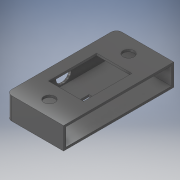
# Autodesk Inventor part: prototype1_third_eye_not_blind
Saved by Autodesk Inventor 2019 (Build 230136000, 136)
## iProperties
Created: 2019-02-05
Part Number: prototype1_third_eye_not_blind
Material: Generic
Document SubType Name: Modeling
Designer: ybharatu
Density: 1 g/cm^3
Appearance: Silicon Nitride - Polished
Author: ybharatu
Autodesk Inventor part; units mm, degrees
ref_plane "YZ Plane" through (0, 0, 0) normal (1, 0, 0) x (0, 1, 0)
ref_plane "XZ Plane" through (0, 0, 0) normal (0, 1, 0) x (-1, 0, 0)
ref_plane "XY Plane" through (0, 0, 0) normal (0, 0, 1) x (1, 0, 0)
sketch "Sketch1" plane through (0, 0, 0) normal (0, 1, 0) x (-1, 0, 0)
  line L0 (122.8458, -138.2757) -> (56.882, -138.2757)
  line L1 (56.882, -138.2757) -> (56.882, -265.2757)
  line L2 (56.882, -265.2757) -> (122.8458, -265.2757)
  line L3 (122.8458, -265.2757) -> (122.8458, -138.2757)
  line L4 (110.1458, -173.9373) -> (69.582, -173.9373)
  line L5 (69.582, -173.9373) -> (69.582, -229.6141)
  line L6 (69.582, -229.6141) -> (110.1458, -229.6141)
  line L7 (110.1458, -229.6141) -> (110.1458, -173.9373)
  point P0 (0, 0)
  dimension "d1" = 127
  dimension "d4" = 55.6768
  dimension "d5" = 40.5638
  dimension "d6" = 12.7
  dimension "d7" = 35.6616
  dimension "d8" = 12.7
  constraints: 16 end point, 4 parallel, 2 horizontal, 2 perpendicular
  measures "d1" distance of L2.end L0.start
  measures "d4" distance of L6.end L4.start
  measures "d5" distance of L5.end L6.end
  measures "d6" distance between parallel lines of L3 L7
  measures "d7" distance between parallel lines of L0 L4
  measures "d8" distance between parallel lines of L5 L1
extrude "Extrusion1" add sketch "Sketch1" along normal blind 25.4 contours L3 L2 L1 L0 | L7 L6 L5 L4
shell "Shell1" thickness 2.54 removed faces 1 at (-56.882, 8.4667, -180.609)
sketch "Sketch3" plane through (0, 25.4, 0) normal (0, 1, 0) x (1, 0, 0)
  line L0 (-110.1458, 174.0389) -> (-69.582, 174.0389)
  line L1 (-69.582, 174.0389) -> (-69.582, 229.7157)
  line L2 (-69.582, 229.7157) -> (-110.1458, 229.7157)
  line L3 (-110.1458, 229.7157) -> (-110.1458, 174.0389)
  line L4 (-122.8458, 265.2757) -> (-122.8458, 138.2757) projected
  line L5 (-56.882, 265.2757) -> (-122.8458, 265.2757) projected
  point P0 (0, 0)
  dimension "d14" = 55.6768
  dimension "d15" = 40.5638
  dimension "d16" = 12.7
  dimension "d17" = 35.56
  constraints: 8 end point, 2 parallel, 1 horizontal, 1 perpendicular
  measures "d14" distance of L2.end L0.start
  measures "d15" distance of L0.start L0.end
  measures "d16" distance between parallel lines of L4 L3
  measures "d17" distance between parallel lines of L5 L2
extrude "Extrusion2" cut sketch "Sketch3" against normal blind 12.7
sketch "Sketch4" plane through (0, 25.4, 0) normal (0, 1, 0) x (1, 0, 0)
  circle A0 centre (-91.0958, 156.2589) radius 6.35
  line L0 (-69.582, 174.0389) -> (-110.1458, 174.0389) projected
  line L1 (-122.8458, 265.2757) -> (-122.8458, 138.2757) projected
  line L2 (-122.8458, 138.2757) -> (-56.882, 138.2757) projected
  line L3 (-69.582, 229.7157) -> (-69.582, 174.0389) projected
  line L4 (-69.582, 174.0389) -> (-110.1458, 174.0389) projected
  line L5 (-110.1458, 174.0389) -> (-110.1458, 229.7157) projected
  line L6 (-110.1458, 229.7157) -> (-69.582, 229.7157) projected
  line L7 (-122.8458, 138.2757) -> (-56.882, 138.2757) projected
  line L8 (-56.882, 138.2757) -> (-56.882, 265.2757) projected
  line L9 (-56.882, 265.2757) -> (-122.8458, 265.2757) projected
  line L10 (-122.8458, 265.2757) -> (-122.8458, 138.2757) projected
  circle A1 centre (-91.0958, 247.4957) radius 6.35
  point P0 (0, 0)
  dimension "d20" = 12.7
  dimension "d21" = 17.78
  dimension "d22" = 31.75
  dimension "d23" = 12.7
  dimension "d24" = 17.78
  dimension "d25" = 31.75
  constraints: 2 centre point
  measures "d20" diameter of A0
  measures "d21" distance from line of L0 A0.centre
  measures "d22" distance from line of L1 A0.centre
  measures "d23" diameter of A1
  measures "d24" distance from line of A1.centre L6
  measures "d25" distance from line of L1 A1.centre
hole "Hole1" at (-91.0958, 25.4, -156.2589) at (-91.0958, 25.4, -247.4957) direction (0, -1, 0) diameter 12.7 depth 12.7 tip angle 118
sketch "Sketch5" plane through (0, 0, 0) normal (0, -1, 0) x (1, 0, 0)
  line L0 (-122.8458, -265.2757) -> (-122.8458, -138.2757) projected
  line L1 (-122.8458, -138.2757) -> (-56.882, -138.2757) projected
  line L2 (-122.8458, -265.2757) -> (-122.8458, -138.2757) projected
  line L3 (-56.882, -265.2757) -> (-122.8458, -265.2757) projected
  line L4 (-56.882, -138.2757) -> (-56.882, -265.2757) projected
  line L5 (-96.1758, -206.8557) -> (-86.0158, -206.8557)
  line L6 (-86.0158, -206.8557) -> (-86.0158, -196.6957)
  line L7 (-86.0158, -196.6957) -> (-96.1758, -196.6957)
  line L8 (-96.1758, -196.6957) -> (-96.1758, -206.8557)
  point P0 (0, 0)
  dimension "d33" = 10.16
  dimension "d34" = 10.16
  dimension "d35" = 26.67
  dimension "d36" = 58.42
  constraints: 8 end point, 2 parallel, 1 horizontal, 1 perpendicular
  measures "d33" distance of L7.end L5.start
  measures "d34" distance of L5.start L5.end
  measures "d35" distance between parallel lines of L0 L8
  measures "d36" distance between parallel lines of L5 L3
extrude "Extrusion3" cut sketch "Sketch5" against normal blind 12.7 contours L8 L7 L6 L5
sketch "Sketch6" plane through (-122.8458, 0, -265.2757) normal (-1, 0, 0) x (0, 0, 1)
  circle A0 centre (63.5, 12.7) radius 8.89
  line L0 (127, 0) -> (127, 25.4) projected
  line L1 (0, 25.4) -> (127, 25.4) projected
  line L2 (116.7244, 19.05) -> (91.3244, 19.05)
  line L3 (91.3244, 19.05) -> (91.3244, 6.35)
  line L4 (91.3244, 6.35) -> (116.7244, 6.35)
  line L5 (116.7244, 6.35) -> (116.7244, 19.05)
  line L6 (0, 0) -> (127, 0) projected
  point P0 (265.2757, 0)
  dimension "d39" = 17.78
  dimension "d40" = 63.5
  dimension "d41" = 12.7
  dimension "d49" = 12.7
  dimension "d50" = 25.4
  dimension "d51" = 6.35
  constraints: 8 end point, 2 parallel, 1 centre point, 1 horizontal, 1 perpendicular
  measures "d39" diameter of A0
  measures "d40" distance from line of L0 A0.centre
  measures "d41" distance from line of L1 A0.centre
  measures "d49" distance of L4.end L2.start
  measures "d50" distance of L2.start L2.end
  measures "d51" distance between parallel lines of L6 L4
hole "Hole2" at (-122.8458, 12.7, -201.7757) direction (1, 0, 0) diameter 17.78 depth 12.7 tip angle 118
extrude "Extrusion4" cut sketch "Sketch6" against normal blind 12.7 contours L5 L4 L3 L2
sketch "Sketch7" plane through (-56.882, 0, -265.2757) normal (0, 0, -1) x (-1, 0, 0)
  circle A0 centre (15.2497, 12.7) radius 2.54
  line L0 (0, 25.4) -> (65.9638, 25.4) projected
  point P0 (-56.882, 0)
  dimension "d54" = 5.08
  dimension "d55" = 12.7
  constraints: 1 centre point
  measures "d54" diameter of A0
  measures "d55" distance from line of L0 A0.centre
hole "Hole3" at (-72.1317, 12.7, -265.2757) direction (0, 0, 1) diameter 5.08 depth 12.7 tip angle 118
fillet "Fillet1" radius 6.35 2 edges at (-122.8458, 12.7, -265.2757) (-122.8458, 12.7, -138.2757)
equation "\"d7\" = -0.5 * d4 + 0.5 * d1"
equation "\"d8\" = d6"
body "Solid1"
